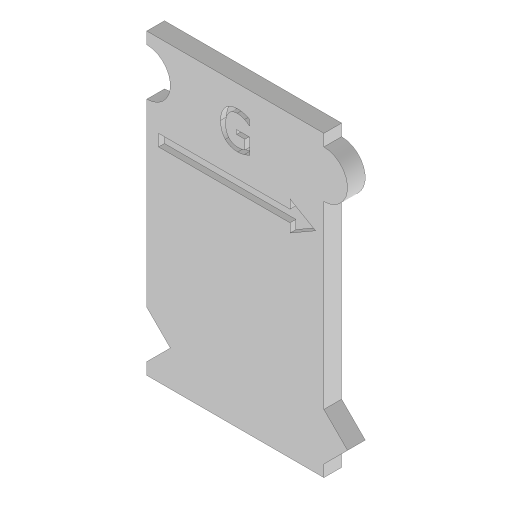
# Autodesk Inventor part: MS_G[202] text
Saved by Autodesk Inventor 2023 (Build 270158000, 158)
## iProperties
Created: 2023-03-29
Part Number: MS_G[202] text
Material: Generic
Document SubType Name: Modeling
Designer: LKLM8608
Density: 1 g/cm^3
Appearance: Default
Author: LKLM8608
Autodesk Inventor part; units mm, degrees
ref_plane "YZ Plane" through (0, 0, 0) normal (1, 0, 0) x (0, 1, 0)
ref_plane "XZ Plane" through (0, 0, 0) normal (0, 1, 0) x (-1, 0, 0)
ref_plane "XY Plane" through (0, 0, 0) normal (0, 0, 1) x (1, 0, 0)
sketch "Sketch1" plane through (0, 0, 0) normal (0, 0, 1) x (1, 0, 0)
  line L0 (-30, 40) -> (0, 40)
  line L1 (-36.1318, 34) -> (13.8682, 34) construction
  arc A0 (0, 30) -> (0, 38) centre (0, 34) ccw
  arc A1 (-30, 30) -> (-30, 38) centre (-30, 34) ccw
  line L2 (-30, 30) -> (0, 30) construction
  line L3 (-30, 0) -> (-30, -4.5) construction
  line L4 (-30, -4.5) -> (0, -4.5) construction
  line L5 (0, -4.5) -> (0, 0) construction
  circle A2 centre (-30, -4.5) radius 4 construction
  circle A3 centre (0, -4.5) radius 4 construction
  line L6 (-30, 0) -> (-30, 30)
  line L7 (-30, 38) -> (-30, 40)
  line L8 (0, 40) -> (0, 38)
  line L9 (0, 30) -> (0, 0)
  line L10 (-30, 0.0688) -> (-30, -0.5)
  line L11 (-30, -0.5) -> (-26, -4.5)
  line L12 (0, 0) -> (0, -0.5)
  line L13 (0, -0.5) -> (4, -4.5)
  line L14 (4, -4.5) -> (0, -8.5)
  line L15 (-26, -4.5) -> (-30, -8.5)
  line L16 (-30, -8.5) -> (-30, -10.5)
  line L17 (-30, -10.5) -> (0, -10.5)
  line L18 (0, -10.5) -> (0, -8.5)
  line L19 (0, 0) -> (-0.5, 0)
  dimension "d0" = 30
  dimension "d1" = 40
  dimension "d2" = 50
  dimension "d3" = 6
  dimension "d4" = 8
  dimension "d5" = 8
  dimension "d6" = 4.5
  dimension "d7" = 8
  dimension "d8" = 8
  dimension "d9" = 2
  constraints: 40 end point, 10 point on circle, 9 point on line, 6 parallel, 6 perpendicular, 4 centre point, 2 coincident, 2 horizontal, 2 vertical
  measures "d0" distance of L0.start L0.end
  measures "d1" distance of L3.start L0.start
  measures "d2" distance of L1.start L1.end
  measures "d3" distance between parallel lines of L1 L0
  measures "d4" diameter of A0
  measures "d5" diameter of A1
  measures "d6" distance of L3.start L3.end
  measures "d7" diameter of A2
  measures "d8" diameter of A3
  measures "d9" distance of L15.end L16.end
extrude "Extrusion1" add sketch "Sketch1" along normal blind 3
sketch "Sketch2" plane through (0, 0, 3) normal (0, 0, 1) x (1, 0, 0)
  line L0 (-30, -10.5) -> (0, -10.5) construction
  line L1 (0, -0.5) -> (0, 30) construction
  line L2 (0, 40) -> (-30, 40) construction
  line L3 (-15, 40) -> (-15, -10.5) construction
  line L4 (-15, 40) -> (-15, 36.5) construction
  line L5 (-15, 36.5) -> (-8.9843, 36.5) construction
  line L6 (-17.7725, 36.2895) -> (-9.6231, 36.2895) construction
  line L7 (-9.6231, 36.2895) -> (-9.6231, 27.3992) construction
  line L8 (-9.6231, 27.3992) -> (-17.7725, 27.3992) construction
  line L9 (-17.7725, 27.3992) -> (-17.7725, 36.2895) construction
  line L10 (-15, -10.5) -> (-15, 26) construction
  line L11 (-15, 26) -> (0, 26) construction
  line L12 (-5.7398, 26) -> (-28, 26)
  line L13 (-28, 26) -> (-28, 24)
  line L14 (-28, 24) -> (-5.7398, 24)
  line L15 (-5.7398, 24) -> (-5.7398, 26)
  line L16 (-28, 25) -> (0, 25) construction
  line L17 (-5.7398, 26) -> (-5.7398, 27.5)
  line L18 (-5.7398, 27.5) -> (-1.4096, 25)
  line L19 (-5.7398, 24) -> (-5.7398, 22.5)
  line L20 (-5.7398, 22.5) -> (-1.4096, 25)
  spline S0 degree 2 poles (-14.5989, 29.9621) (-15.2464, 29.9621) (-16.3191, 30.3575) (-16.7047, 30.7579) knots 0 0 0 1 2 2 2
  spline S1 degree 2 poles (-16.7047, 30.7579) (-17.0903, 31.1633) (-17.5006, 32.3596) (-17.5006, 33.1357) knots 0 0 0 1 2 2 2
  spline S2 degree 2 poles (-17.5006, 33.1357) (-17.5006, 33.8722) (-17.0853, 35.0388) (-16.6998, 35.4541) knots 0 0 0 1 2 2 2
  spline S3 degree 2 poles (-16.6998, 35.4541) (-16.329, 35.8545) (-15.2415, 36.2895) (-14.5939, 36.2895) knots 0 0 0 1 2 2 2
  spline S4 degree 2 poles (-14.5939, 36.2895) (-14.2825, 36.2895) (-13.719, 36.2005) (-13.4619, 36.1214) knots 0 0 0 1 2 2 2
  spline S5 degree 2 poles (-13.4619, 36.1214) (-13.2543, 36.0621) (-12.7501, 35.8446) (-12.5969, 35.7655) knots 0 0 0 1 2 2 2
  line L21 (-12.5969, 35.7655) -> (-12.5969, 34.7867)
  line L22 (-12.5969, 34.7867) -> (-12.6661, 34.7867)
  spline S6 degree 2 poles (-12.6661, 34.7867) (-12.8193, 34.9202) (-13.1406, 35.1624) (-13.4372, 35.3008) knots 0 0 0 1 2 2 2
  spline S7 degree 2 poles (-13.4372, 35.3008) (-13.6844, 35.4244) (-14.3221, 35.5875) (-14.6879, 35.5875) knots 0 0 0 1 2 2 2
  spline S8 degree 2 poles (-14.6879, 35.5875) (-15.5678, 35.5875) (-16.6553, 34.2627) (-16.6553, 33.1604) knots 0 0 0 1 2 2 2
  spline S9 degree 2 poles (-16.6553, 33.1604) (-16.6553, 32.5474) (-16.3686, 31.628) (-16.0967, 31.3116) knots 0 0 0 1 2 2 2
  spline S10 degree 2 poles (-16.0967, 31.3116) (-15.8347, 30.9952) (-15.0932, 30.664) (-14.6285, 30.664) knots 0 0 0 1 2 2 2
  spline S11 degree 2 poles (-14.6285, 30.664) (-14.2875, 30.664) (-13.6053, 30.7629) (-13.3729, 30.8618) knots 0 0 0 1 2 2 2
  line L23 (-13.3729, 30.8618) -> (-13.3729, 32.4387)
  line L24 (-13.3729, 32.4387) -> (-14.7867, 32.4387)
  line L25 (-14.7867, 32.4387) -> (-14.7867, 33.1505)
  line L26 (-14.7867, 33.1505) -> (-12.5721, 33.1505)
  line L27 (-12.5721, 33.1505) -> (-12.5721, 30.4861)
  spline S12 degree 2 poles (-12.5721, 30.4861) (-12.7254, 30.4169) (-13.2494, 30.2043) (-13.4718, 30.14) knots 0 0 0 1 2 2 2
  spline S13 degree 2 poles (-13.4718, 30.14) (-13.7734, 30.0511) (-14.2578, 29.9621) (-14.5989, 29.9621) knots 0 0 0 1 2 2 2
  point P0 (0, 0)
  dimension "d12" = 3.5
  dimension "d13" = 36.5
  dimension "d14" = 2
  dimension "d15" = 1.5
  dimension "d16" = 5
  dimension "d17" = 1.5
  dimension "d58" = 14
  constraints: 28 end point, 7 point on line, 3 midpoint, 3 perpendicular, 2 horizontal, 2 parallel, 1 vertical, 2 other
  measures "d12" distance of L3.start L4.end
  measures "d13" distance of L3.end L10.end
  measures "d14" distance of L13.end L12.end
  measures "d15" distance of L12.start L17.end
  measures "d16" distance of L17.end L18.end
  measures "d17" distance of L14.end L19.end
  measures "d58" distance between parallel lines of L2 L12
extrude "Extrusion2" cut sketch "Sketch2" against normal blind 1
sketch "Sketch5" plane through (0, 0, 0) normal (0, 0, -1) x (-1, 0, 0)
  line L0 (30, 30) -> (30, -0.5) construction
  arc A0 (30, 38) -> (30, 30) centre (30, 34) ccw construction
  line L1 (30, 40) -> (30, 38) construction
  line L2 (0, 40) -> (30, 40) construction
  line L3 (0, 38) -> (0, 40) construction
  arc A1 (0, 38) -> (0, 30) centre (0, 34) ccw construction
  line L4 (0, -0.5) -> (0, 30) construction
  line L5 (-4, -4.5) -> (0, -0.5) construction
  line L6 (0, -8.5) -> (-4, -4.5) construction
  line L7 (0, -10.5) -> (0, -8.5) construction
  line L8 (30, -10.5) -> (0, -10.5) construction
  line L9 (30, -8.5) -> (30, -10.5) construction
  line L10 (26, -4.5) -> (30, -8.5) construction
  line L11 (30, -0.5) -> (26, -4.5) construction
  point P0 (0, 0)
sketch "Sketch6" plane through (0, 0, 0) normal (0, 0, -1) x (-1, 0, 0)
  line L0 (30, 30) -> (30, -0.5) construction
  line L1 (0, 40) -> (30, 40) construction
  line L2 (30, -10.5) -> (0, -10.5) construction
  line L3 (17.9728, -6.9957) -> (10.1851, -6.9957) construction
  line L4 (10.1851, -6.9957) -> (10.1851, 2.1518) construction
  line L5 (10.1851, 2.1518) -> (17.9728, 2.1518) construction
  line L6 (17.9728, 2.1518) -> (17.9728, -6.9957) construction
  line L7 (15, -10.5) -> (15, 40) construction
  line L8 (15, -10.5) -> (15, -7) construction
  line L9 (15, -7) -> (11.2598, -7) construction
  line L10 (16.564, 40) -> (16.564, 4) construction
  line L11 (16.564, 4) -> (24.4907, 4) construction
  line L12 (30, 5.5) -> (28, 5.5) construction
  line L13 (28, 5.5) -> (6.5, 5.5)
  line L14 (6.5, 5.5) -> (6.5, 3.5)
  line L15 (6.5, 3.5) -> (28, 3.5)
  line L16 (28, 3.5) -> (28, 5.5)
  line L17 (6.5, 3.5) -> (6.5, 2)
  line L18 (6.5, 2) -> (2.1699, 4.5)
  line L19 (6.5, 5.5) -> (6.5, 7)
  line L20 (6.5, 7) -> (2.1699, 4.5)
  line L21 (5.7398, 24) -> (28, 24) construction
  line L22 (28, 26) -> (5.7398, 26) construction
  line L23 (1.1699, 23) -> (6.1699, 23)
  line L24 (6.1699, 23) -> (6.1699, 25)
  line L25 (6.1699, 25) -> (1.1699, 25)
  line L26 (1.1699, 25) -> (1.1699, 23)
  line L27 (7.1699, 23) -> (12.1699, 23)
  line L28 (12.1699, 25) -> (7.1699, 25)
  line L29 (12.1699, 23) -> (12.1699, 25)
  line L30 (7.1699, 25) -> (7.1699, 23)
  line L31 (13.1699, 23) -> (18.1699, 23)
  line L32 (18.1699, 25) -> (13.1699, 25)
  line L33 (18.1699, 23) -> (18.1699, 25)
  line L34 (13.1699, 25) -> (13.1699, 23)
  line L35 (19.1699, 23) -> (24.1699, 23)
  line L36 (24.1699, 25) -> (19.1699, 25)
  line L37 (24.1699, 23) -> (24.1699, 25)
  line L38 (19.1699, 25) -> (19.1699, 23)
  line L39 (24.1699, 23) -> (24.1699, 21.5)
  line L40 (24.1699, 21.5) -> (28.635, 23.75)
  line L41 (24.1699, 25) -> (24.1699, 26.5)
  line L42 (24.1699, 26.5) -> (28.635, 23.75)
  line L43 (0, -0.5) -> (0, 30) construction
  line L44 (28, 4.5) -> (0, 4.5) construction
  spline S0 degree 2 poles (14.7992, -0.6683) (15.4468, -0.6683) (16.5195, -1.0638) (16.9051, -1.4642) knots 0 0 0 1 2 2 2
  spline S1 degree 2 poles (16.9051, -1.4642) (17.2906, -1.8695) (17.7009, -3.0658) (17.7009, -3.8419) knots 0 0 0 1 2 2 2
  spline S2 degree 2 poles (17.7009, -3.8419) (17.7009, -4.5784) (17.2857, -5.745) (16.9001, -6.1603) knots 0 0 0 1 2 2 2
  spline S3 degree 2 poles (16.9001, -6.1603) (16.5294, -6.5607) (15.4419, -6.9957) (14.7943, -6.9957) knots 0 0 0 1 2 2 2
  spline S4 degree 2 poles (14.7943, -6.9957) (14.4829, -6.9957) (13.9193, -6.9067) (13.6623, -6.8276) knots 0 0 0 1 2 2 2
  spline S5 degree 2 poles (13.6623, -6.8276) (13.4547, -6.7683) (12.9505, -6.5508) (12.7972, -6.4717) knots 0 0 0 1 2 2 2
  line L45 (12.7972, -6.4717) -> (12.7972, -5.4929)
  line L46 (12.7972, -5.4929) -> (12.8664, -5.4929)
  spline S6 degree 2 poles (12.8664, -5.4929) (13.0197, -5.6264) (13.341, -5.8686) (13.6376, -6.007) knots 0 0 0 1 2 2 2
  spline S7 degree 2 poles (13.6376, -6.007) (13.8847, -6.1306) (14.5224, -6.2937) (14.8882, -6.2937) knots 0 0 0 1 2 2 2
  spline S8 degree 2 poles (14.8882, -6.2937) (15.7681, -6.2937) (16.8556, -4.9689) (16.8556, -3.8666) knots 0 0 0 1 2 2 2
  spline S9 degree 2 poles (16.8556, -3.8666) (16.8556, -3.2536) (16.5689, -2.3342) (16.2971, -2.0178) knots 0 0 0 1 2 2 2
  spline S10 degree 2 poles (16.2971, -2.0178) (16.0351, -1.7014) (15.2936, -1.3702) (14.8289, -1.3702) knots 0 0 0 1 2 2 2
  spline S11 degree 2 poles (14.8289, -1.3702) (14.4878, -1.3702) (13.8056, -1.4691) (13.5733, -1.568) knots 0 0 0 1 2 2 2
  line L47 (13.5733, -1.568) -> (13.5733, -3.1449)
  line L48 (13.5733, -3.1449) -> (14.9871, -3.1449)
  line L49 (14.9871, -3.1449) -> (14.9871, -3.8567)
  line L50 (14.9871, -3.8567) -> (12.7725, -3.8567)
  line L51 (12.7725, -3.8567) -> (12.7725, -1.1923)
  spline S12 degree 2 poles (12.7725, -1.1923) (12.9257, -1.1231) (13.4497, -0.9105) (13.6722, -0.8462) knots 0 0 0 1 2 2 2
  spline S13 degree 2 poles (13.6722, -0.8462) (13.9737, -0.7573) (14.4582, -0.6683) (14.7992, -0.6683) knots 0 0 0 1 2 2 2
  point P0 (0, 0)
  dimension "d36" = 3.5
  dimension "d37" = 36
  dimension "d38" = 2
  dimension "d39" = 1.5
  dimension "d40" = 5
  dimension "d41" = 1.5
  dimension "d42" = 5
  dimension "d43" = 2
  dimension "d46" = 6
  dimension "d51" = 1.5
  dimension "d52" = 5
  dimension "d53" = 1.5
  dimension "d56" = 18.5
  dimension "d57" = 14
  constraints: 70 end point, 7 perpendicular, 5 point on line, 4 parallel, 4 vertical, 3 horizontal, 3 midpoint, 26 other
  measures "d36" distance of L7.start L8.end
  measures "d37" distance of L10.start L10.end
  measures "d38" distance of L14.end L13.end
  measures "d39" distance of L14.end L17.end
  measures "d40" distance of L17.end L18.end
  measures "d41" distance of L13.end L19.end
  measures "d42" distance of L25.end L24.end
  measures "d43" distance of L24.end L23.end
  measures "d46" distance of L23.end L27.end
  measures "d51" distance of L35.end L39.end
  measures "d52" distance of L39.end L40.end
  measures "d53" distance of L36.start L41.end
  measures "d56" distance from line of L1 L39.end
  measures "d57" distance between parallel lines of L15 L2
extrude "Extrusion4" cut sketch "Sketch6" against normal blind 1
body "Solid1"
